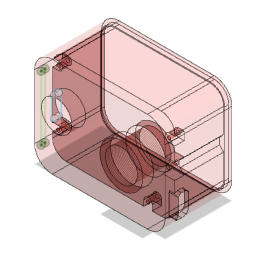
MDCEnclosure (Autodesk Fusion 360 design; units mm, degrees)
Autodesk Fusion 360 part; units mm, degrees
(part 1 of 2)
sketch "BackplateMountPoint" plane through (0, 0, 0) normal (0, 0, 1) x (1, 0, 0)
  line L0 (44.005, 19.075) -> (42.505, 17.575)
  line L1 (42.505, 17.575) -> (42.505, 15.075)
  line L2 (42.505, 15.075) -> (44.005, 13.575)
  line L3 (44.005, 13.575) -> (44.005, 19.075)
  line L4 (44.005, 16.325) -> (42.505, 16.325) construction
  line L5 (44.005, 4.75) -> (44.005, 27.9)
  point P0 (43.905, 16.325)
  dimension "d514" = 1.5
  dimension "d515" = 135
  dimension "d516" = 135
  dimension "d517" = 2.5
  dimension "d518" = 0.1
  constraint midpoint L3 L4.start
  constraint coincident L4 P0
  constraint midpoint L3 L5
  measures "d514" distance of L1 L3
  measures "d515" angle of L0 L1
  measures "d516" angle of L1 L2
  measures "d517" distance of L0.end L1.end
  measures "d518" distance of L3 P0
sketch "Board" plane through (0, 0, 0) normal (0, 0, 1) x (1, 0, 0)
  line L0 (4.75, 0) -> (39.105, 0)
  line L1 (43.855, 4.75) -> (43.855, 27.9)
  line L2 (39.105, 32.65) -> (4.75, 32.65)
  line L3 (0, 27.9) -> (0, 4.75)
  arc A0 (4.75, 32.65) -> (0, 27.9) centre (4.75, 27.9) ccw
  arc A1 (43.855, 27.9) -> (39.105, 32.65) centre (39.105, 27.9) ccw
  arc A2 (39.105, 0) -> (43.855, 4.75) centre (39.105, 4.75) ccw
  arc A3 (0, 4.75) -> (4.75, 0) centre (4.75, 4.75) ccw
  line L4 (-0.15, 27.9) -> (-0.15, 4.75)
  arc A4 (-0.15, 4.75) -> (4.75, -0.15) centre (4.75, 4.75) ccw
  line L5 (4.75, -0.15) -> (39.105, -0.15)
  arc A5 (39.105, -0.15) -> (44.005, 4.75) centre (39.105, 4.75) ccw
  line L6 (44.005, 4.75) -> (44.005, 27.9)
  arc A6 (44.005, 27.9) -> (39.105, 32.8) centre (39.105, 27.9) ccw
  line L7 (39.105, 32.8) -> (4.75, 32.8)
  arc A7 (4.75, 32.8) -> (-0.15, 27.9) centre (4.75, 27.9) ccw
  line L8 (-0.35, 27.9) -> (-0.35, 4.75)
  arc A8 (-0.35, 4.75) -> (4.75, -0.35) centre (4.75, 4.75) ccw
  line L9 (4.75, -0.35) -> (39.105, -0.35)
  arc A9 (39.105, -0.35) -> (44.205, 4.75) centre (39.105, 4.75) ccw
  line L10 (44.205, 4.75) -> (44.205, 27.9)
  arc A10 (44.205, 27.9) -> (39.105, 33) centre (39.105, 27.9) ccw
  line L11 (39.105, 33) -> (4.75, 33)
  arc A11 (4.75, 33) -> (-0.35, 27.9) centre (4.75, 27.9) ccw
  line L12 (-0.5, 27.9) -> (-0.5, 4.75)
  arc A12 (-0.5, 4.75) -> (4.75, -0.5) centre (4.75, 4.75) ccw
  line L13 (4.75, -0.5) -> (39.105, -0.5)
  arc A13 (39.105, -0.5) -> (44.355, 4.75) centre (39.105, 4.75) ccw
  line L14 (44.355, 4.75) -> (44.355, 27.9)
  arc A14 (44.355, 27.9) -> (39.105, 33.15) centre (39.105, 27.9) ccw
  line L15 (39.105, 33.15) -> (4.75, 33.15)
  arc A15 (4.75, 33.15) -> (-0.5, 27.9) centre (4.75, 27.9) ccw
  line L16 (21.9275, 32.65) -> (21.9275, 0)
  point P0 (21.9275, 16.325)
  dimension "d329" = 43.855
  dimension "d330" = 32.65
  dimension "d331" = 4.75
  dimension "d332" = 0.15
  dimension "d336" = 0.35
  dimension "d337" = 0.5
  constraint horizontal L0
  constraint vertical L1
  constraint horizontal L2
  constraint vertical L3
  constraint tangent L2 A0
  constraint tangent L3 A0
  constraint tangent L1 A1
  constraint tangent L2 A1
  constraint equal A0 A1
  constraint tangent L0 A2
  constraint tangent L1 A2
  constraint equal A0 A2
  constraint tangent L0 A3
  constraint tangent L3 A3
  constraint equal A0 A3
  constraint midpoint L2 L16.start
  constraint midpoint L0 L16.end
  constraint midpoint L16 P0
  measures "d329" distance of L1 L3
  measures "d330" distance of L0 L2
  measures "d331" radius of A0
sketch "MountPoints" plane through (0, 0, 0) normal (0, 0, 1) x (1, 0, 0)
  line L0 (-0.15, 29.9) -> (0.44, 29.9)
  line L1 (0.44, 29.9) -> (0.44, 26.9)
  line L2 (0.44, 26.9) -> (-0.15, 26.9)
  line L3 (-0.15, 26.9) -> (-0.15, 29.9)
  line L4 (0.44, 29.9) -> (1.94, 29.9)
  line L5 (3.44, 28.4) -> (3.44, 28.4)
  line L6 (1.94, 26.9) -> (0.44, 26.9)
  line L7 (0.44, 26.9) -> (0.44, 29.9)
  line L8 (43.472, 27.333) -> (44.005, 27.333)
  line L9 (44.005, 27.333) -> (44.005, 24.333)
  line L10 (44.005, 24.333) -> (43.472, 24.333)
  line L11 (43.472, 24.333) -> (43.472, 27.333)
  line L12 (41.972, 27.333) -> (43.472, 27.333)
  line L13 (43.472, 27.333) -> (43.472, 24.333)
  line L14 (43.472, 24.333) -> (41.972, 24.333)
  line L15 (40.472, 25.833) -> (40.472, 25.833)
  line L16 (34.3061, 3.4078) -> (34.3065, 3.4078)
  line L17 (35.8063, 1.9078) -> (35.8063, 0.4078)
  line L18 (35.8063, 0.4078) -> (32.8063, 0.4078)
  line L19 (32.8063, 0.4078) -> (32.8063, 1.9078)
  line L20 (32.8063, 0.4078) -> (35.8063, 0.4078)
  line L21 (35.8063, 0.4078) -> (35.8063, -0.15)
  line L22 (35.8063, -0.15) -> (32.8063, -0.15)
  line L23 (32.8063, -0.15) -> (32.8063, 0.4078)
  line L24 (0.39, 9.672) -> (1.89, 9.672)
  line L25 (3.39, 8.172) -> (3.39, 8.172)
  line L26 (1.89, 6.672) -> (0.39, 6.672)
  line L27 (0.39, 6.672) -> (0.39, 9.672)
  line L28 (-0.15, 9.672) -> (0.39, 9.672)
  line L29 (0.39, 9.672) -> (0.39, 6.672)
  line L30 (0.39, 6.672) -> (-0.15, 6.672)
  line L31 (-0.15, 6.672) -> (-0.15, 9.672)
  line L32 (-0.15, 27.9) -> (-0.15, 4.75)
  line L33 (44.005, 4.75) -> (44.005, 27.9)
  line L34 (4.75, -0.15) -> (39.105, -0.15)
  line L35 (0.44, 28.4) -> (3.44, 28.4) construction
  line L36 (40.472, 25.833) -> (43.472, 25.833) construction
  line L37 (32.8063, 1.9078) -> (35.8063, 1.9078) construction
  line L38 (0.39, 8.172) -> (3.39, 8.172) construction
  line L39 (0, 27.9) -> (0, 4.75) construction
  line L40 (4.75, 0) -> (39.105, 0) construction
  arc A0 (3.44, 28.4) -> (1.94, 29.9) centre (1.94, 28.4) ccw
  arc A1 (1.94, 26.9) -> (3.44, 28.4) centre (1.94, 28.4) ccw
  arc A2 (41.972, 27.333) -> (40.472, 25.833) centre (41.972, 25.833) ccw
  arc A3 (40.472, 25.833) -> (41.972, 24.333) centre (41.972, 25.833) ccw
  arc A4 (34.3061, 3.4078) -> (32.8063, 1.9078) centre (34.3063, 1.9078) ccw
  arc A5 (35.8063, 1.9078) -> (34.3065, 3.4078) centre (34.3063, 1.9078) ccw
  arc A6 (3.39, 8.172) -> (1.89, 9.672) centre (1.89, 8.172) ccw
  arc A7 (1.89, 6.672) -> (3.39, 8.172) centre (1.89, 8.172) ccw
  line L41 (44.005, 19.175) -> (39.505, 19.175)
  line L42 (39.505, 19.175) -> (39.505, 13.475)
  line L43 (39.505, 13.475) -> (44.005, 13.475)
  line L44 (44.005, 13.475) -> (44.005, 19.175)
  line L45 (44.005, 4.75) -> (44.005, 27.9)
  line L46 (44.005, 13.575) -> (44.005, 19.075)
  line L47 (44.005, 16.325) -> (39.505, 16.325)
  point P0 (1.94, 28.4)
  point P1 (41.972, 25.833)
  point P2 (34.3063, 1.9078)
  point P3 (1.89, 8.172)
  point P4 (44.005, 19.075)
  point P5 (41.505, 16.325)
  dimension "d404" = 3
  dimension "d407" = 3
  dimension "d409" = 3
  dimension "d411" = 3
  dimension "d412" = 1.89
  dimension "d413" = 8.172
  dimension "d414" = 34.3063
  dimension "d415" = 1.9078
  dimension "d416" = 41.972
  dimension "d417" = 25.833
  dimension "d418" = 1.94
  dimension "d419" = 28.4
  dimension "d422" = 1.5
  dimension "d566" = 0.1
  dimension "d567" = 4.5
  dimension "d568" = 2.5
  constraint horizontal L0
  constraint vertical L1
  constraint horizontal L2
  constraint vertical L3
  constraint horizontal L4
  constraint horizontal L6
  constraint vertical L7
  constraint horizontal L8
  constraint vertical L9
  constraint horizontal L10
  constraint vertical L11
  constraint horizontal L12
  constraint vertical L13
  constraint horizontal L14
  constraint vertical L17
  constraint horizontal L18
  constraint vertical L19
  constraint horizontal L20
  constraint vertical L21
  constraint horizontal L22
  constraint vertical L23
  constraint horizontal L24
  constraint horizontal L26
  constraint vertical L27
  constraint horizontal L28
  constraint vertical L29
  constraint horizontal L30
  constraint vertical L31
  constraint collinear L1 L7
  constraint collinear L0 L4
  constraint collinear L2 L6
  constraint collinear L3 L32
  constraint collinear L11 L13
  constraint collinear L9 L33
  constraint collinear L8 L12
  constraint collinear L10 L14
  constraint collinear L18 L20
  constraint collinear L22 L34
  constraint collinear L19 L23
  constraint collinear L17 L21
  constraint collinear L27 L29
  constraint collinear L24 L28
  constraint collinear L26 L30
  constraint collinear L31 L32
  constraint midpoint L1 L35.start
  constraint midpoint L13 L36.end
  constraint midpoint L29 L38.start
  constraint midpoint L35 P0
  constraint midpoint L36 P1
  constraint midpoint L37 P2
  constraint midpoint L38 P3
  constraint tangent L4 A0
  constraint tangent L6 A1
  constraint equal A0 A1
  constraint tangent L12 A2
  constraint equal A0 A2
  constraint tangent L14 A3
  constraint equal A0 A3
  constraint coincident L19 L37.start
  constraint tangent L19 A4
  constraint equal A0 A4
  constraint coincident L17 L37.end
  constraint tangent L17 A5
  constraint equal A0 A5
  constraint tangent L24 A6
  constraint equal A0 A6
  constraint tangent L26 A7
  constraint equal A0 A7
  constraint horizontal L41
  constraint vertical L42
  constraint horizontal L43
  constraint vertical L44
  constraint midpoint L44 L45
  constraint midpoint L46 L47.start
  constraint midpoint L42 L47.end
  constraint coincident L47 P5
  measures "d404" distance of L4 L6
  measures "d407" distance of L12 L14
  measures "d409" distance of L17 L19
  measures "d411" distance of L24 L26
  measures "d412" distance of P3 L39
  measures "d413" distance of P3 L40
  measures "d414" distance of P2 L39
  measures "d415" distance of P2 L40
  measures "d416" distance of P1 L39
  measures "d417" distance of P1 L40
  measures "d418" distance of P0 L39
  measures "d419" distance of P0 L40
  measures "d422" radius of A0
  measures "d566" distance of L41 P4
  measures "d567" distance of L42 L46
  measures "d568" distance of L44 P5
extrude "Front-Sidewalls" add sketch "Board" along normal blind 24.16 thin wall 1.5 on the left open curves L4 A4 L5 A5 L6 A6 L7 A7 makes body 1 in component "Front"
sketch "FrontHoles" plane through (0, 0, 0) normal (0, 0, 1) x (1, 0, 0)
  line L0 (0, 27.9) -> (0, 4.75)
  line L1 (4.75, 0) -> (39.105, 0)
  circle A0 centre (33.5424, 17.392) radius 7.2644
  circle A1 centre (33.5424, 17.392) radius 7.7644
  point P0 (6.2926, 17.392)
  point P1 (33.5424, 17.392)
  dimension "d350" = 6.2926
  dimension "d351" = 17.392
  dimension "d352" = 33.5424
  dimension "d353" = 17.392
  dimension "d554" = 14.5287
  dimension "d555" = 15.5287
  measures "d350" distance of P0 L0
  measures "d351" distance of P0 L1
  measures "d352" distance of P1 L0
  measures "d353" distance of P1 L1
  measures "d554" diameter of A0
  measures "d555" diameter of A1
extrude "Front-Frontplate" add sketch "Board" along normal blind 5 separate body contours L0 L2 L3 A0 A3 L16 | L0 L1 L2 A1 A2 L16 | L4 A4 L5 A5 L6 A6 L7 A7 makes body 2 in component "Front"
hole "Front-MotionSensorHole" at (6.2926, 17.392, 0) direction (0, 0, 1) diameter 11 depth 12 tip angle 118 bodies 2 in component "Front"
extrude "Front-LensProtrusionInside" [suppressed]
extrude "Extrude12" add sketch "FrontHoles" against normal blind 3.36 contours A0 bodies 2 in component "Front"
extrude "Front-LensProtrusionOutside" [suppressed]
extrude "Extrude13" add sketch "FrontHoles" along normal blind 8.84 contours A0 | A1 bodies 2 in component "Front"
hole "Hole8" at (33.5424, 17.392, -3.36) direction (0, 0, 1) diameter 11.529 end through all bodies 1 2 in component "Front"
thread "Thread2" "ISO Metric profile 12.0 M12x0.5 6H" major diameter 12.0961 minor diameter 11.5287 pitch 0.5 angle 60 resizes the face on face at (33.8297, 23.1493, 0.7067) on bodies 2 in component "Front"
copy_body "Body->Comp3" bodies 2 removing the originals makes body 3 in component "Component"
extrude "Front-BoardMountPoints" add sketch "MountPoints" against normal blind 3.36 separate body contours L0 L1 L2 L3 L7 L32 | L1 L4 L6 L7 A0 A1 | L8 L9 L10 L11 L13 L33 L45 | L11 L12 L13 L14 A2 A3 | L17 L18 L19 L20 A4 A5 | L18 L20 L21 L22 L23 L34 | L24 L26 L27 L29 A6 A7 | L27 L28 L29 L30 L31 L32 makes body 4 at (3.0647, 27.4075, -1.12) makes body 5 at (3.3895, 8.1346, -2.24) makes body 6 at (41.1898, 27.1129, -2.24) makes body 7 at (34.8063, -0.15, -1.12) in component "Component"
hole "Front-BoardMountPointHoles" at (41.972, 25.833, 0) at (1.94, 28.4, 0) at (1.89, 8.172, 0) at (34.3063, 1.9078, 0) direction (0, 0, -1) diameter 1.3 depth 3.36 tip angle 180 bodies 4 5 6 7 in component "Component"
extrude "Front-BackplateInset" cut sketch "Board" along normal blind 1.5 contours L0 L2 L3 A0 A3 L16 | L0 L1 L2 A1 A2 L16 | L4 A4 L5 A5 L6 A6 L7 A7 | L8 A8 L9 A9 L10 A10 L11 A11 | L12 A12 L13 A13 L14 A14 L15 A15 bodies 1 in component "Front"
extrude "Front-BackplateMountPoint" add sketch "BackplateMountPoint" along normal blind 19.16 from surface at 1.5 bodies 1 in component "Front"
move_body "Front-FrontplateAlign" bodies 6 4 3 7 5 to x (1, 0, 0) y (0, 1, 0) z (0, 0, 1) at (0, 0, 19.16) in component "Component"
extrude "Front-BackplateMountPointExtrude" add sketch "MountPoints" along normal blind 3.36 separate body contours L33 L42 L43 L44 L45 L46 L47 | L33 L41 L42 L44 L45 L46 L47 makes body 8 in component "Front"
hole "Hole9" at (41.505, 16.325, 0) direction (0, 0, 1) diameter 1.271 depth 3.36 tip angle 180 bodies 8 in component "Front"
thread "Thread3" "ISO Metric profile 1.6 M1.6x0.35 6H" in component "Front"
move_body "Front-BackplateMountPointAlign" bodies 8 to x (1, 0, 0) y (0, 1, 0) z (0, 0, 1) at (0, 0, 15.8) in component "Front"
combine "Front-Combine" operation add target body 1 tool bodies 3 4 7 5 6 8 in component "Front"
extrude "Back-Backplate" add sketch "Board" along normal blind 1.5 separate body contours L0 L2 L3 A0 A3 L16 | L0 L1 L2 A1 A2 L16 | L4 A4 L5 A5 L6 A6 L7 A7 | L8 A8 L9 A9 L10 A10 L11 A11 makes body 9 in component "Back"
sketch "HoleSemicircleTool" plane through (0, 0, 0) normal (0, 0, 1) x (1, 0, 0) in component "Back"
  line L0 (-2.65, 16.975) -> (-0.05, 16.975)
  line L1 (-0.05, 16.975) -> (-0.05, 15.675)
  line L2 (-0.05, 15.675) -> (-2.65, 15.675)
  line L3 (-2.65, 15.675) -> (-2.65, 16.975)
  point P0 (-0.05, 16.325)
  dimension "d509" = 1.3
  dimension "d510" = 2.6
  constraint horizontal L0
  constraint vertical L1
  constraint horizontal L2
  constraint vertical L3
  constraint midpoint L1 P0
  measures "d509" distance of L0 L2
  measures "d510" distance of L1 L3
extrude "Extrude3" cut sketch "HoleSemicircleTool" along normal blind 1.5 bodies 9 in component "Back"
sketch "Sketch1" plane through (0, 0, 0) normal (0, 0, 1) x (1, 0, 0) in component "Battery"
  line L0 (20, 15) -> (-20, 15)
  line L1 (-20, 15) -> (-20, -15)
  line L2 (-20, -15) -> (20, -15)
  line L3 (20, -15) -> (20, 15)
  line L4 (20, 15) -> (-20, -15) construction
  dimension "d443" = 40
  dimension "d444" = 30
  constraint horizontal L0
  constraint vertical L1
  constraint horizontal L2
  constraint vertical L3
  constraint midpoint L4 origin
  measures "d443" distance of L1 L3
  measures "d444" distance of L0 L2
extrude "Extrude1" add sketch "Sketch1" along normal blind 11.2 separate body makes body 10 in component "Battery"
move_body "Align1" bodies 10 to x (1, 0, 0) y (0, 1, 0) z (0, 0, 1) at (21.9275, 16.325, 1.5) in component "Battery"
ref_plane "WorkPlane3" through (21.9275, 16.325, 12.08) normal (1, 0, 0) x (0, 1, 0) in component "Front"
sketch "BackplateScrewHeadInset" plane through (0, 0, 0) normal (0, 0, 1) x (1, 0, 0)
  line L0 (0.45, 17.825) -> (-10.05, 17.825)
  line L1 (-10.05, 17.825) -> (-10.05, 14.825)
  line L2 (-10.05, 14.825) -> (0.45, 14.825)
  line L3 (1.45, 15.825) -> (1.45, 16.825)
  line L4 (1.45, 16.325) -> (-10.05, 16.325)
  arc A0 (1.45, 16.825) -> (0.45, 17.825) centre (0.45, 16.825) ccw
  arc A1 (0.45, 14.825) -> (1.45, 15.825) centre (0.45, 15.825) ccw
  point P0 (-0.05, 16.325)
  point P1 (-0.05, 16.325)
  dimension "d461" = 3
  dimension "d462" = 1.5
  dimension "d463" = 1
  dimension "d464" = 10
  constraint horizontal L0
  constraint vertical L1
  constraint horizontal L2
  constraint vertical L3
  constraint midpoint L1 L4.end
  constraint coincident L4 P1
  constraint coincident L3 L4.start
  constraint tangent L0 A0
  constraint tangent L3 A0
  constraint tangent L2 A1
  constraint tangent L3 A1
  constraint equal A0 A1
  constraint coincident P1 P0
  measures "d461" distance of L0 L2
  measures "d462" distance of L3 P1
  measures "d463" radius of A0
  measures "d464" distance of L1 P1
extrude "Extrude1'" add sketch "Board" along normal blind 3.1 separate body contours L0 L2 L3 A0 A3 L16 | L0 L1 L2 A1 A2 L16 makes body 11 in component "Board"
move_body "Align1'" bodies 11 to x (1, 0, 0) y (0, 1, 0) z (0, 0, 1) at (0, 0, 12.7) in component "Board"
sketch "USBCPlugCutout" plane through (0, 0, 0) normal (1, 0, 0) x (0, 0, -1) in component "Front"
  line L0 (-22, 4.75) -> (-22, 27.9)
  line L1 (-22, 27.9) -> (-23.5, 27.9)
  line L2 (-23.5, 27.9) -> (-23.5, 4.75)
  line L3 (-23.5, 4.75) -> (-22, 4.75)
  line L4 (-18.715, 19.0109) -> (-17.155, 19.0109)
  line L5 (-16.155, 18.0109) -> (-16.155, 10.6709)
  line L6 (-17.155, 9.6709) -> (-18.715, 9.6709)
  line L7 (-19.715, 10.6709) -> (-19.715, 18.0109)
  arc A0 (-18.715, 19.0109) -> (-19.715, 18.0109) centre (-18.715, 18.0109) ccw
  arc A1 (-16.155, 18.0109) -> (-17.155, 19.0109) centre (-17.155, 18.0109) ccw
  arc A2 (-17.155, 9.6709) -> (-16.155, 10.6709) centre (-17.155, 10.6709) ccw
  arc A3 (-19.715, 10.6709) -> (-18.715, 9.6709) centre (-18.715, 10.6709) ccw
  dimension "d492" = 3.56
  dimension "d493" = 9.34
  dimension "d497" = 1
  dimension "d498" = 1
  dimension "d499" = 1
  constraint horizontal L4
  constraint vertical L5
  constraint vertical L7
  constraint tangent L4 A0
  constraint tangent L7 A0
  constraint tangent L4 A1
  constraint tangent L5 A1
  constraint tangent L5 A2
  constraint tangent L6 A2
  constraint tangent L6 A3
  constraint tangent L7 A3
  constraint equal A2 A3
  measures "d492" distance of L5 L7
  measures "d493" distance of L4 L6
  measures "d497" radius of A0
  measures "d498" radius of A1
  measures "d499" radius of A2
extrude "Extrude9" add sketch "USBCPlugCutout" along normal blind 10 separate body contours L4 L5 L6 L7 A0 A1 A2 A3 makes body 12 in component "Front"
ref_plane "WorkPlane5" through (34.3063, 1.6289, 15.7) normal (0, 0, -1) x (-1, 0, 0) in component "Front"
ref_plane "WorkPlane6" through (42.005, 16.325, 21.66) normal (1, 0, 0) x (0, 1, 0) in component "Front"
move_body "Align3" bodies 12 to x (1, 0, 0) y (0, 1, 0) z (0, 0, 1) at (42.005, 0, 0) in component "Front"
move_body "Align4" bodies 12 to x (1, 0, 0) y (0, 1, 0) z (0, 0, 1) at (0, 0, -0.455) in component "Front"
ref_plane "WorkPlane7" through (21.9275, 0, 0) normal (0, -1, 0) x (1, 0, 0) in component "Front"
ref_plane "WorkPlane9" through (21.9275, 5.2535, 0) normal (0, -1, 0) x (1, 0, 0) in component "Front"
move_body "Align5" bodies 12 to x (1, 0, 0) y (0, 1, 0) z (0, 0, 1) at (0, -9.0874, 0) in component "Front"
combine "Combine3" operation cut target body 1 tool bodies 12 in component "Front"
sketch "MDC" plane through (0, 0, 0) normal (0, 0, 1) x (1, 0, 0) in component "PCB"
  arc A0 (41.5, 32.002) -> (39.105, 32.65) centre (39.105, 27.9) ccw
  line L0 (39.105, 32.65) -> (4.75, 32.65)
  arc A1 (39.105, 0) -> (43.855, 4.75) centre (39.105, 4.75) ccw
  line L1 (0, 27.9) -> (0, 4.75)
  line L2 (43.855, 4.75) -> (43.855, 27.94)
  arc A2 (0, 4.75) -> (4.75, 0) centre (4.75, 4.75) ccw
  circle A3 centre (33.5424, 26.392) radius 0.85
  line L3 (41.5, 27.94) -> (41.5, 32.002)
  line L4 (4.75, 0) -> (39.105, 0)
  line L5 (41.5, 27.94) -> (43.855, 27.94)
  arc A4 (4.75, 32.65) -> (0, 27.9) centre (4.75, 27.9) ccw
  circle A5 centre (33.5424, 8.392) radius 0.85
  circle A6 centre (31.327, 4.655) radius 0.4953
  arc A7 (20.7054, 5.534) -> (20.7054, 5.7626) centre (20.7054, 5.6483) ccw
  arc A8 (20.7054, 5.534) -> (20.7054, 5.7626) centre (20.7054, 5.6483) ccw
  arc A9 (20.7054, 5.7626) -> (20.7054, 5.534) centre (20.7054, 5.6483) ccw
  arc A10 (20.7054, 5.7626) -> (20.7054, 5.534) centre (20.7054, 5.6483) ccw
  arc A11 (25.253, 5.5373) -> (25.253, 5.7659) centre (25.253, 5.6516) ccw
  arc A12 (25.253, 5.7659) -> (25.253, 5.5373) centre (25.253, 5.6516) ccw
  arc A13 (24.6078, 4.8871) -> (24.6078, 5.1157) centre (24.6078, 5.0014) ccw
  arc A14 (21.5834, 17.8471) -> (21.5834, 18.0757) centre (21.5834, 17.9614) ccw
  arc A15 (1.89, 8.922) -> (1.89, 7.422) centre (1.89, 8.172) ccw
  arc A16 (21.5834, 17.8471) -> (21.5834, 18.0757) centre (21.5834, 17.9614) ccw
  arc A17 (21.5834, 18.0757) -> (21.5834, 17.8471) centre (21.5834, 17.9614) ccw
  arc A18 (21.5834, 17.0597) -> (21.5834, 17.2883) centre (21.5834, 17.174) ccw
  arc A19 (21.5834, 18.0757) -> (21.5834, 17.8471) centre (21.5834, 17.9614) ccw
  arc A20 (20.7706, 17.0597) -> (20.7706, 17.2883) centre (20.7706, 17.174) ccw
  arc A21 (20.7706, 17.2883) -> (20.7706, 17.0597) centre (20.7706, 17.174) ccw
  arc A22 (20.7706, 16.2469) -> (20.7706, 16.4755) centre (20.7706, 16.3612) ccw
  arc A23 (21.5834, 17.2883) -> (21.5834, 17.0597) centre (21.5834, 17.174) ccw
  arc A24 (21.5834, 17.2883) -> (21.5834, 17.0597) centre (21.5834, 17.174) ccw
  arc A25 (21.5834, 17.0597) -> (21.5834, 17.2883) centre (21.5834, 17.174) ccw
  arc A26 (25.2581, 4.8896) -> (25.2581, 5.1182) centre (25.2581, 5.0039) ccw
  arc A27 (25.2581, 5.1182) -> (25.2581, 4.8896) centre (25.2581, 5.0039) ccw
  arc A28 (25.2581, 4.8896) -> (25.2581, 5.1182) centre (25.2581, 5.0039) ccw
  arc A29 (20.7706, 17.2883) -> (20.7706, 17.0597) centre (20.7706, 17.174) ccw
  arc A30 (20.7706, 17.0597) -> (20.7706, 17.2883) centre (20.7706, 17.174) ccw
  arc A31 (20.7706, 16.4755) -> (20.7706, 16.2469) centre (20.7706, 16.3612) ccw
  arc A32 (21.3566, 4.2368) -> (21.3566, 4.4654) centre (21.3566, 4.3511) ccw
  arc A33 (21.3566, 4.4654) -> (21.3566, 4.2368) centre (21.3566, 4.3511) ccw
  arc A34 (21.3566, 4.2368) -> (21.3566, 4.4654) centre (21.3566, 4.3511) ccw
  arc A35 (20.7706, 16.4755) -> (20.7706, 16.2469) centre (20.7706, 16.3612) ccw
  arc A36 (20.7706, 16.2469) -> (20.7706, 16.4755) centre (20.7706, 16.3612) ccw
  arc A37 (25.2581, 5.1182) -> (25.2581, 4.8896) centre (25.2581, 5.0039) ccw
  arc A38 (10.8138, 28.8136) -> (10.8138, 29.1057) centre (10.8138, 28.9596) ccw
  arc A39 (10.8138, 29.1057) -> (10.8138, 28.8136) centre (10.8138, 28.9596) ccw
  arc A40 (11.2431, 28.364) -> (11.2431, 28.6561) centre (11.2431, 28.51) ccw
  arc A41 (25.253, 5.7659) -> (25.253, 5.5373) centre (25.253, 5.6516) ccw
  arc A42 (25.253, 5.5373) -> (25.253, 5.7659) centre (25.253, 5.6516) ccw
  arc A43 (24.6078, 5.1157) -> (24.6078, 4.8871) centre (24.6078, 5.0014) ccw
  arc A44 (14.5578, 25.1534) -> (14.5578, 25.4455) centre (14.5578, 25.2995) ccw
  arc A45 (14.5578, 25.4455) -> (14.5578, 25.1534) centre (14.5578, 25.2995) ccw
  arc A46 (14.5578, 25.1534) -> (14.5578, 25.4455) centre (14.5578, 25.2995) ccw
  arc A47 (24.6078, 5.1157) -> (24.6078, 4.8871) centre (24.6078, 5.0014) ccw
  arc A48 (24.6078, 4.8871) -> (24.6078, 5.1157) centre (24.6078, 5.0014) ccw
  arc A49 (21.3566, 4.4654) -> (21.3566, 4.2368) centre (21.3566, 4.3511) ccw
  arc A50 (15.0556, 24.6988) -> (15.0556, 24.9908) centre (15.0556, 24.8448) ccw
  arc A51 (15.0556, 24.9908) -> (15.0556, 24.6988) centre (15.0556, 24.8448) ccw
  arc A52 (9.0891, 27.1804) -> (9.0891, 27.4724) centre (9.0891, 27.3264) ccw
  arc A53 (10.8138, 29.1057) -> (10.8138, 28.8136) centre (10.8138, 28.9596) ccw
  arc A54 (10.8138, 28.8136) -> (10.8138, 29.1057) centre (10.8138, 28.9596) ccw
  arc A55 (11.2431, 28.6561) -> (11.2431, 28.364) centre (11.2431, 28.51) ccw
  arc A56 (10.0569, 25.617) -> (10.0569, 25.8456) centre (10.0569, 25.7313) ccw
  arc A57 (10.0569, 25.8456) -> (10.0569, 25.617) centre (10.0569, 25.7313) ccw
  arc A58 (10.0569, 25.617) -> (10.0569, 25.8456) centre (10.0569, 25.7313) ccw
  arc A59 (11.2431, 28.6561) -> (11.2431, 28.364) centre (11.2431, 28.51) ccw
  arc A60 (11.2431, 28.364) -> (11.2431, 28.6561) centre (11.2431, 28.51) ccw
  arc A61 (14.5578, 25.4455) -> (14.5578, 25.1534) centre (14.5578, 25.2995) ccw
  arc A62 (11.1999, 24.479) -> (11.1999, 24.7076) centre (11.1999, 24.5933) ccw
  arc A63 (11.1999, 24.7076) -> (11.1999, 24.479) centre (11.1999, 24.5933) ccw
  arc A64 (12.8864, 21.6444) -> (12.8864, 21.873) centre (12.8864, 21.7587) ccw
  arc A65 (15.0556, 24.9908) -> (15.0556, 24.6988) centre (15.0556, 24.8448) ccw
  arc A66 (15.0556, 24.6988) -> (15.0556, 24.9908) centre (15.0556, 24.8448) ccw
  arc A67 (9.0891, 27.4724) -> (9.0891, 27.1804) centre (9.0891, 27.3264) ccw
  arc A68 (12.287, 28.9977) -> (12.287, 29.2263) centre (12.287, 29.112) ccw
  arc A69 (12.287, 29.2263) -> (12.287, 28.9977) centre (12.287, 29.112) ccw
  arc A70 (12.287, 28.9977) -> (12.287, 29.2263) centre (12.287, 29.112) ccw
  arc A71 (9.0891, 27.4724) -> (9.0891, 27.1804) centre (9.0891, 27.3264) ccw
  arc A72 (9.0891, 27.1804) -> (9.0891, 27.4724) centre (9.0891, 27.3264) ccw
  arc A73 (10.0569, 25.8456) -> (10.0569, 25.617) centre (10.0569, 25.7313) ccw
  arc A74 (13.4452, 27.8572) -> (13.4452, 28.0858) centre (13.4452, 27.9715) ccw
  arc A75 (13.4452, 28.0858) -> (13.4452, 27.8572) centre (13.4452, 27.9715) ccw
  arc A76 (12.2819, 24.446) -> (12.2819, 24.6746) centre (12.2819, 24.5603) ccw
  arc A77 (11.1999, 24.7076) -> (11.1999, 24.479) centre (11.1999, 24.5933) ccw
  arc A78 (11.1999, 24.479) -> (11.1999, 24.7076) centre (11.1999, 24.5933) ccw
  arc A79 (12.8864, 21.873) -> (12.8864, 21.6444) centre (12.8864, 21.7587) ccw
  arc A80 (14.0371, 26.2012) -> (14.0371, 26.4298) centre (14.0371, 26.3155) ccw
  arc A81 (14.0371, 26.4298) -> (14.0371, 26.2012) centre (14.0371, 26.3155) ccw
  arc A82 (14.0371, 26.2012) -> (14.0371, 26.4298) centre (14.0371, 26.3155) ccw
  arc A83 (12.8864, 21.873) -> (12.8864, 21.6444) centre (12.8864, 21.7587) ccw
  arc A84 (12.8864, 21.6444) -> (12.8864, 21.873) centre (12.8864, 21.7587) ccw
  arc A85 (12.287, 29.2263) -> (12.287, 28.9977) centre (12.287, 29.112) ccw
  arc A86 (6.9597, 9.5923) -> (6.9597, 9.8845) centre (6.9597, 9.7384) ccw
  arc A87 (6.9597, 9.8845) -> (6.9597, 9.5923) centre (6.9597, 9.7384) ccw
  arc A88 (6.9466, 8.9396) -> (6.9466, 9.2316) centre (6.9466, 9.0856) ccw
  arc A89 (13.4452, 28.0858) -> (13.4452, 27.8572) centre (13.4452, 27.9715) ccw
  arc A90 (13.4452, 27.8572) -> (13.4452, 28.0858) centre (13.4452, 27.9715) ccw
  arc A91 (12.2819, 24.6746) -> (12.2819, 24.446) centre (12.2819, 24.5603) ccw
  arc A92 (4.3625, 26.4779) -> (4.3625, 26.77) centre (4.3625, 26.6239) ccw
  arc A93 (4.3625, 26.77) -> (4.3625, 26.4779) centre (4.3625, 26.6239) ccw
  arc A94 (4.3625, 26.4779) -> (4.3625, 26.77) centre (4.3625, 26.6239) ccw
  arc A95 (12.2819, 24.6746) -> (12.2819, 24.446) centre (12.2819, 24.5603) ccw
  arc A96 (12.2819, 24.446) -> (12.2819, 24.6746) centre (12.2819, 24.5603) ccw
  arc A97 (14.0371, 26.4298) -> (14.0371, 26.2012) centre (14.0371, 26.3155) ccw
  arc A98 (19.6911, 6.487) -> (19.6911, 6.779) centre (19.6911, 6.633) ccw
  arc A99 (19.6911, 6.779) -> (19.6911, 6.487) centre (19.6911, 6.633) ccw
  arc A100 (23.9481, 7.1169) -> (23.9481, 7.409) centre (23.9481, 7.2629) ccw
  arc A101 (6.9597, 9.8845) -> (6.9597, 9.5923) centre (6.9597, 9.7384) ccw
  arc A102 (6.9597, 9.5923) -> (6.9597, 9.8845) centre (6.9597, 9.7384) ccw
  arc A103 (6.9466, 9.2316) -> (6.9466, 8.9396) centre (6.9466, 9.0856) ccw
  arc A104 (27.7556, 13.3538) -> (27.7556, 13.5824) centre (27.7556, 13.4681) ccw
  arc A105 (27.7556, 13.5824) -> (27.7556, 13.3538) centre (27.7556, 13.4681) ccw
  arc A106 (27.7556, 13.3538) -> (27.7556, 13.5824) centre (27.7556, 13.4681) ccw
  arc A107 (6.9466, 9.2316) -> (6.9466, 8.9396) centre (6.9466, 9.0856) ccw
  arc A108 (6.9466, 8.9396) -> (6.9466, 9.2316) centre (6.9466, 9.0856) ccw
  arc A109 (4.3625, 26.77) -> (4.3625, 26.4779) centre (4.3625, 26.6239) ccw
  arc A110 (27.7454, 12.6452) -> (27.7454, 12.8738) centre (27.7454, 12.7595) ccw
  arc A111 (27.7454, 12.8738) -> (27.7454, 12.6452) centre (27.7454, 12.7595) ccw
  arc A112 (17.8394, 3.8517) -> (17.8394, 4.0803) centre (17.8394, 3.966) ccw
  arc A113 (19.6911, 6.779) -> (19.6911, 6.487) centre (19.6911, 6.633) ccw
  arc A114 (19.6911, 6.487) -> (19.6911, 6.779) centre (19.6911, 6.633) ccw
  arc A115 (23.9481, 7.409) -> (23.9481, 7.1169) centre (23.9481, 7.2629) ccw
  arc A116 (20.7655, 15.4747) -> (20.7655, 15.7033) centre (20.7655, 15.589) ccw
  arc A117 (20.7655, 15.7033) -> (20.7655, 15.4747) centre (20.7655, 15.589) ccw
  arc A118 (20.7655, 15.4747) -> (20.7655, 15.7033) centre (20.7655, 15.589) ccw
  arc A119 (23.9481, 7.409) -> (23.9481, 7.1169) centre (23.9481, 7.2629) ccw
  arc A120 (23.9481, 7.1169) -> (23.9481, 7.409) centre (23.9481, 7.2629) ccw
  arc A121 (27.7556, 13.5824) -> (27.7556, 13.3538) centre (27.7556, 13.4681) ccw
  arc A122 (13.4275, 22.2235) -> (13.4275, 22.4521) centre (13.4275, 22.3378) ccw
  arc A123 (13.4275, 22.4521) -> (13.4275, 22.2235) centre (13.4275, 22.3378) ccw
  arc A124 (16.8893, 2.2531) -> (16.8893, 2.4817) centre (16.8893, 2.3674) ccw
  arc A125 (27.7454, 12.8738) -> (27.7454, 12.6452) centre (27.7454, 12.7595) ccw
  arc A126 (27.7454, 12.6452) -> (27.7454, 12.8738) centre (27.7454, 12.7595) ccw
  arc A127 (17.8394, 4.0803) -> (17.8394, 3.8517) centre (17.8394, 3.966) ccw
  arc A128 (16.8893, 5.5334) -> (16.8893, 5.762) centre (16.8893, 5.6477) ccw
  arc A129 (16.8893, 5.762) -> (16.8893, 5.5334) centre (16.8893, 5.6477) ccw
  arc A130 (16.8893, 5.5334) -> (16.8893, 5.762) centre (16.8893, 5.6477) ccw
  arc A131 (17.8394, 4.0803) -> (17.8394, 3.8517) centre (17.8394, 3.966) ccw
  arc A132 (17.8394, 3.8517) -> (17.8394, 4.0803) centre (17.8394, 3.966) ccw
  arc A133 (20.7655, 15.7033) -> (20.7655, 15.4747) centre (20.7655, 15.589) ccw
  arc A134 (11.4969, 5.912) -> (11.4969, 6.204) centre (11.4969, 6.058) ccw
  arc A135 (11.4969, 6.204) -> (11.4969, 5.912) centre (11.4969, 6.058) ccw
  arc A136 (28.543, 12.456) -> (28.543, 12.7481) centre (28.543, 12.602) ccw
  arc A137 (13.4275, 22.4521) -> (13.4275, 22.2235) centre (13.4275, 22.3378) ccw
  arc A138 (13.4275, 22.2235) -> (13.4275, 22.4521) centre (13.4275, 22.3378) ccw
  arc A139 (16.8893, 2.4817) -> (16.8893, 2.2531) centre (16.8893, 2.3674) ccw
  arc A140 (26.1224, 10.2514) -> (26.1224, 10.48) centre (26.1224, 10.3657) ccw
  arc A141 (26.1224, 10.48) -> (26.1224, 10.2514) centre (26.1224, 10.3657) ccw
  arc A142 (26.1224, 10.2514) -> (26.1224, 10.48) centre (26.1224, 10.3657) ccw
  arc A143 (16.8893, 2.4817) -> (16.8893, 2.2531) centre (16.8893, 2.3674) ccw
  arc A144 (16.8893, 2.2531) -> (16.8893, 2.4817) centre (16.8893, 2.3674) ccw
  arc A145 (16.8893, 5.762) -> (16.8893, 5.5334) centre (16.8893, 5.6477) ccw
  arc A146 (27.1333, 27.8155) -> (27.1333, 28.0441) centre (27.1333, 27.9298) ccw
  arc A147 (27.1333, 28.0441) -> (27.1333, 27.8155) centre (27.1333, 27.9298) ccw
  arc A148 (28.9011, 30.0711) -> (28.9011, 30.2997) centre (28.9011, 30.1854) ccw
  arc A149 (11.4969, 6.204) -> (11.4969, 5.912) centre (11.4969, 6.058) ccw
  arc A150 (11.4969, 5.912) -> (11.4969, 6.204) centre (11.4969, 6.058) ccw
  arc A151 (28.543, 12.7481) -> (28.543, 12.456) centre (28.543, 12.602) ccw
  arc A152 (28.416, 14.1097) -> (28.416, 14.3383) centre (28.416, 14.224) ccw
  arc A153 (28.416, 14.3383) -> (28.416, 14.1097) centre (28.416, 14.224) ccw
  arc A154 (28.416, 14.1097) -> (28.416, 14.3383) centre (28.416, 14.224) ccw
  arc A155 (28.543, 12.7481) -> (28.543, 12.456) centre (28.543, 12.602) ccw
  arc A156 (28.543, 12.456) -> (28.543, 12.7481) centre (28.543, 12.602) ccw
  arc A157 (26.1224, 10.48) -> (26.1224, 10.2514) centre (26.1224, 10.3657) ccw
  arc A158 (6.2824, 4.5644) -> (6.2824, 4.793) centre (6.2824, 4.6787) ccw
  arc A159 (6.2824, 4.793) -> (6.2824, 4.5644) centre (6.2824, 4.6787) ccw
  arc A160 (6.2824, 2.1844) -> (6.2824, 2.413) centre (6.2824, 2.2987) ccw
  arc A161 (27.1333, 28.0441) -> (27.1333, 27.8155) centre (27.1333, 27.9298) ccw
  arc A162 (27.1333, 27.8155) -> (27.1333, 28.0441) centre (27.1333, 27.9298) ccw
  arc A163 (28.9011, 30.2997) -> (28.9011, 30.0711) centre (28.9011, 30.1854) ccw
  arc A164 (27.2212, 19.0045) -> (27.2212, 19.2965) centre (27.2212, 19.1505) ccw
  arc A165 (27.2212, 19.2965) -> (27.2212, 19.0045) centre (27.2212, 19.1505) ccw
  arc A166 (27.2212, 19.0045) -> (27.2212, 19.2965) centre (27.2212, 19.1505) ccw
  arc A167 (28.9011, 30.2997) -> (28.9011, 30.0711) centre (28.9011, 30.1854) ccw
  arc A168 (28.9011, 30.0711) -> (28.9011, 30.2997) centre (28.9011, 30.1854) ccw
  arc A169 (28.416, 14.3383) -> (28.416, 14.1097) centre (28.416, 14.224) ccw
  arc A170 (18.51, 10.0457) -> (18.51, 10.2743) centre (18.51, 10.16) ccw
  arc A171 (18.51, 10.2743) -> (18.51, 10.0457) centre (18.51, 10.16) ccw
  arc A172 (17.9182, 6.2459) -> (17.9182, 6.4745) centre (17.9182, 6.3602) ccw
  arc A173 (6.2824, 4.793) -> (6.2824, 4.5644) centre (6.2824, 4.6787) ccw
  arc A174 (6.2824, 4.5644) -> (6.2824, 4.793) centre (6.2824, 4.6787) ccw
  arc A175 (6.2824, 2.413) -> (6.2824, 2.1844) centre (6.2824, 2.2987) ccw
  arc A176 (33.1074, 14.8996) -> (33.1074, 15.1282) centre (33.1074, 15.0139) ccw
  arc A177 (33.1074, 15.1282) -> (33.1074, 14.8996) centre (33.1074, 15.0139) ccw
  arc A178 (33.1074, 14.8996) -> (33.1074, 15.1282) centre (33.1074, 15.0139) ccw
  arc A179 (6.2824, 2.413) -> (6.2824, 2.1844) centre (6.2824, 2.2987) ccw
  arc A180 (6.2824, 2.1844) -> (6.2824, 2.413) centre (6.2824, 2.2987) ccw
  arc A181 (27.2212, 19.2965) -> (27.2212, 19.0045) centre (27.2212, 19.1505) ccw
  arc A182 (36.1224, 31.6954) -> (36.1224, 31.9874) centre (36.1224, 31.8414) ccw
  arc A183 (36.1224, 31.9874) -> (36.1224, 31.6954) centre (36.1224, 31.8414) ccw
  arc A184 (34.7609, 31.8846) -> (34.7609, 32.1132) centre (34.7609, 31.9989) ccw
  arc A185 (18.51, 10.2743) -> (18.51, 10.0457) centre (18.51, 10.16) ccw
  arc A186 (18.51, 10.0457) -> (18.51, 10.2743) centre (18.51, 10.16) ccw
  arc A187 (17.9182, 6.4745) -> (17.9182, 6.2459) centre (17.9182, 6.3602) ccw
  arc A188 (28.1849, 20.6654) -> (28.1849, 20.894) centre (28.1849, 20.7797) ccw
  arc A189 (28.1849, 20.894) -> (28.1849, 20.6654) centre (28.1849, 20.7797) ccw
  arc A190 (28.1849, 20.6654) -> (28.1849, 20.894) centre (28.1849, 20.7797) ccw
  arc A191 (17.9182, 6.4745) -> (17.9182, 6.2459) centre (17.9182, 6.3602) ccw
  arc A192 (17.9182, 6.2459) -> (17.9182, 6.4745) centre (17.9182, 6.3602) ccw
  arc A193 (33.1074, 15.1282) -> (33.1074, 14.8996) centre (33.1074, 15.0139) ccw
  arc A194 (29.526, 21.3563) -> (29.526, 21.5849) centre (29.526, 21.4706) ccw
  arc A195 (29.526, 21.5849) -> (29.526, 21.3563) centre (29.526, 21.4706) ccw
  arc A196 (30.2448, 4.0259) -> (30.2448, 4.2545) centre (30.2448, 4.1402) ccw
  arc A197 (36.1224, 31.9874) -> (36.1224, 31.6954) centre (36.1224, 31.8414) ccw
  arc A198 (36.1224, 31.6954) -> (36.1224, 31.9874) centre (36.1224, 31.8414) ccw
  arc A199 (34.7609, 32.1132) -> (34.7609, 31.8846) centre (34.7609, 31.9989) ccw
  arc A200 (30.0518, 2.601) -> (30.0518, 2.8296) centre (30.0518, 2.7153) ccw
  arc A201 (30.0518, 2.8296) -> (30.0518, 2.601) centre (30.0518, 2.7153) ccw
  arc A202 (30.0518, 2.601) -> (30.0518, 2.8296) centre (30.0518, 2.7153) ccw
  arc A203 (34.7609, 32.1132) -> (34.7609, 31.8846) centre (34.7609, 31.9989) ccw
  arc A204 (34.7609, 31.8846) -> (34.7609, 32.1132) centre (34.7609, 31.9989) ccw
  arc A205 (28.1849, 20.894) -> (28.1849, 20.6654) centre (28.1849, 20.7797) ccw
  arc A206 (13.2852, 6.2763) -> (13.2852, 6.5049) centre (13.2852, 6.3906) ccw
  arc A207 (13.2852, 6.5049) -> (13.2852, 6.2763) centre (13.2852, 6.3906) ccw
  arc A208 (12.7417, 5.4381) -> (12.7417, 5.6667) centre (12.7417, 5.5524) ccw
  arc A209 (29.526, 21.5849) -> (29.526, 21.3563) centre (29.526, 21.4706) ccw
  arc A210 (29.526, 21.3563) -> (29.526, 21.5849) centre (29.526, 21.4706) ccw
  arc A211 (30.2448, 4.2545) -> (30.2448, 4.0259) centre (30.2448, 4.1402) ccw
  arc A212 (9.7419, 5.9563) -> (9.7419, 6.1849) centre (9.7419, 6.0706) ccw
  arc A213 (9.7419, 6.1849) -> (9.7419, 5.9563) centre (9.7419, 6.0706) ccw
  arc A214 (9.7419, 5.9563) -> (9.7419, 6.1849) centre (9.7419, 6.0706) ccw
  arc A215 (30.2448, 4.2545) -> (30.2448, 4.0259) centre (30.2448, 4.1402) ccw
  arc A216 (30.2448, 4.0259) -> (30.2448, 4.2545) centre (30.2448, 4.1402) ccw
  arc A217 (30.0518, 2.8296) -> (30.0518, 2.601) centre (30.0518, 2.7153) ccw
  arc A218 (24.7508, 19.4437) -> (24.7508, 19.6723) centre (24.7508, 19.558) ccw
  arc A219 (24.7508, 19.6723) -> (24.7508, 19.4437) centre (24.7508, 19.558) ccw
  arc A220 (28.731, 23.4467) -> (28.731, 23.6753) centre (28.731, 23.561) ccw
  arc A221 (13.2852, 6.5049) -> (13.2852, 6.2763) centre (13.2852, 6.3906) ccw
  arc A222 (13.2852, 6.2763) -> (13.2852, 6.5049) centre (13.2852, 6.3906) ccw
  arc A223 (12.7417, 5.6667) -> (12.7417, 5.4381) centre (12.7417, 5.5524) ccw
  arc A224 (34.5222, 5.1392) -> (34.5222, 5.3678) centre (34.5222, 5.2535) ccw
  arc A225 (34.5222, 5.3678) -> (34.5222, 5.1392) centre (34.5222, 5.2535) ccw
  arc A226 (34.5222, 5.1392) -> (34.5222, 5.3678) centre (34.5222, 5.2535) ccw
  arc A227 (12.7417, 5.6667) -> (12.7417, 5.4381) centre (12.7417, 5.5524) ccw
  arc A228 (12.7417, 5.4381) -> (12.7417, 5.6667) centre (12.7417, 5.5524) ccw
  arc A229 (9.7419, 6.1849) -> (9.7419, 5.9563) centre (9.7419, 6.0706) ccw
  arc A230 (26.4983, 24.3916) -> (26.4983, 24.6202) centre (26.4983, 24.5059) ccw
  arc A231 (26.4983, 24.6202) -> (26.4983, 24.3916) centre (26.4983, 24.5059) ccw
  arc A232 (23.91, 28.9826) -> (23.91, 29.2747) centre (23.91, 29.1287) ccw
  arc A233 (24.7508, 19.6723) -> (24.7508, 19.4437) centre (24.7508, 19.558) ccw
  arc A234 (24.7508, 19.4437) -> (24.7508, 19.6723) centre (24.7508, 19.558) ccw
  arc A235 (28.731, 23.6753) -> (28.731, 23.4467) centre (28.731, 23.561) ccw
  arc A236 (32.226, 28.556) -> (32.226, 28.8481) centre (32.226, 28.702) ccw
  arc A237 (32.226, 28.8481) -> (32.226, 28.556) centre (32.226, 28.702) ccw
  arc A238 (32.226, 28.556) -> (32.226, 28.8481) centre (32.226, 28.702) ccw
  arc A239 (28.731, 23.6753) -> (28.731, 23.4467) centre (28.731, 23.561) ccw
  arc A240 (28.731, 23.4467) -> (28.731, 23.6753) centre (28.731, 23.561) ccw
  arc A241 (34.5222, 5.3678) -> (34.5222, 5.1392) centre (34.5222, 5.2535) ccw
  arc A242 (28.7919, 26.3601) -> (28.7919, 26.5887) centre (28.7919, 26.4744) ccw
  arc A243 (28.7919, 26.5887) -> (28.7919, 26.3601) centre (28.7919, 26.4744) ccw
  arc A244 (36.29, 13.5699) -> (36.29, 13.862) centre (36.29, 13.716) ccw
  arc A245 (26.4983, 24.6202) -> (26.4983, 24.3916) centre (26.4983, 24.5059) ccw
  arc A246 (26.4983, 24.3916) -> (26.4983, 24.6202) centre (26.4983, 24.5059) ccw
  arc A247 (23.91, 29.2747) -> (23.91, 28.9826) centre (23.91, 29.1287) ccw
  arc A248 (36.29, 12.808) -> (36.29, 13.1) centre (36.29, 12.954) ccw
  arc A249 (36.29, 13.1) -> (36.29, 12.808) centre (36.29, 12.954) ccw
  arc A250 (36.29, 12.808) -> (36.29, 13.1) centre (36.29, 12.954) ccw
  arc A251 (23.91, 29.2747) -> (23.91, 28.9826) centre (23.91, 29.1287) ccw
  arc A252 (23.91, 28.9826) -> (23.91, 29.2747) centre (23.91, 29.1287) ccw
  arc A253 (32.226, 28.8481) -> (32.226, 28.556) centre (32.226, 28.702) ccw
  arc A254 (30.9306, 16.7869) -> (30.9306, 17.0155) centre (30.9306, 16.9012) ccw
  arc A255 (30.9306, 17.0155) -> (30.9306, 16.7869) centre (30.9306, 16.9012) ccw
  arc A256 (28.7919, 26.5887) -> (28.7919, 26.3601) centre (28.7919, 26.4744) ccw
  arc A257 (28.7919, 26.3601) -> (28.7919, 26.5887) centre (28.7919, 26.4744) ccw
  arc A258 (36.29, 13.862) -> (36.29, 13.5699) centre (36.29, 13.716) ccw
  arc A259 (10.6858, 8.7122) -> (10.6858, 8.9408) centre (10.6858, 8.8265) ccw
  arc A260 (10.6858, 8.9408) -> (10.6858, 8.7122) centre (10.6858, 8.8265) ccw
  arc A261 (36.29, 13.862) -> (36.29, 13.5699) centre (36.29, 13.716) ccw
  arc A262 (36.29, 13.5699) -> (36.29, 13.862) centre (36.29, 13.716) ccw
  arc A263 (36.29, 13.1) -> (36.29, 12.808) centre (36.29, 12.954) ccw
  arc A264 (1.89, 7.422) -> (1.89, 8.922) centre (1.89, 8.172) ccw
  arc A265 (1.89, 7.422) -> (1.89, 8.922) centre (1.89, 8.172) ccw
  arc A266 (30.9306, 17.0155) -> (30.9306, 16.7869) centre (30.9306, 16.9012) ccw
  arc A267 (30.9306, 16.7869) -> (30.9306, 17.0155) centre (30.9306, 16.9012) ccw
  arc A268 (1.94, 27.65) -> (1.94, 29.15) centre (1.94, 28.4) ccw
  arc A269 (1.94, 27.65) -> (1.94, 29.15) centre (1.94, 28.4) ccw
  arc A270 (1.89, 8.922) -> (1.89, 7.422) centre (1.89, 8.172) ccw
  arc A271 (1.94, 29.15) -> (1.94, 27.65) centre (1.94, 28.4) ccw
  arc A272 (41.7272, 10.9338) -> (41.7272, 11.2104) centre (41.7272, 11.0721) ccw
  arc A273 (34.3063, 1.1578) -> (34.3063, 2.6578) centre (34.3063, 1.9078) ccw
  arc A274 (34.3063, 1.1578) -> (34.3063, 2.6578) centre (34.3063, 1.9078) ccw
  arc A275 (41.972, 25.083) -> (41.972, 26.583) centre (41.972, 25.833) ccw
  arc A276 (1.94, 29.15) -> (1.94, 27.65) centre (1.94, 28.4) ccw
  arc A277 (41.972, 25.083) -> (41.972, 26.583) centre (41.972, 25.833) ccw
  arc A278 (41.7272, 11.2104) -> (41.7272, 10.9338) centre (41.7272, 11.0721) ccw
  arc A279 (41.7272, 11.2104) -> (41.7272, 10.9338) centre (41.7272, 11.0721) ccw
  arc A280 (39.5249, 2.2377) -> (39.5249, 2.4663) centre (39.5249, 2.352) ccw
  arc A281 (41.7272, 10.9338) -> (41.7272, 11.2104) centre (41.7272, 11.0721) ccw
  arc A282 (41.972, 26.583) -> (41.972, 25.083) centre (41.972, 25.833) ccw
  arc A283 (41.972, 26.583) -> (41.972, 25.083) centre (41.972, 25.833) ccw
  arc A284 (34.3063, 2.6578) -> (34.3063, 1.1578) centre (34.3063, 1.9078) ccw
  arc A285 (34.3063, 2.6578) -> (34.3063, 1.1578) centre (34.3063, 1.9078) ccw
  arc A286 (39.5249, 2.4663) -> (39.5249, 2.2377) centre (39.5249, 2.352) ccw
  arc A287 (10.6858, 8.7122) -> (10.6858, 8.9408) centre (10.6858, 8.8265) ccw
  arc A288 (39.5249, 2.4663) -> (39.5249, 2.2377) centre (39.5249, 2.352) ccw
  arc A289 (39.5249, 2.2377) -> (39.5249, 2.4663) centre (39.5249, 2.352) ccw
  arc A290 (10.6858, 8.9408) -> (10.6858, 8.7122) centre (10.6858, 8.8265) ccw
  arc A291 (21.6783, 12.2455) -> (21.6783, 12.4741) centre (21.6783, 12.3598) ccw
  arc A292 (21.6783, 12.2455) -> (21.6783, 12.4741) centre (21.6783, 12.3598) ccw
  arc A293 (21.6783, 12.4741) -> (21.6783, 12.2455) centre (21.6783, 12.3598) ccw
  arc A294 (21.6783, 11.6486) -> (21.6783, 11.8772) centre (21.6783, 11.7629) ccw
  arc A295 (21.6783, 12.4741) -> (21.6783, 12.2455) centre (21.6783, 12.3598) ccw
  arc A296 (21.6783, 11.8772) -> (21.6783, 11.6486) centre (21.6783, 11.7629) ccw
  arc A297 (21.6783, 11.8772) -> (21.6783, 11.6486) centre (21.6783, 11.7629) ccw
  arc A298 (21.6783, 11.6486) -> (21.6783, 11.8772) centre (21.6783, 11.7629) ccw
  arc A299 (20.7554, 19.4752) -> (20.7554, 19.7038) centre (20.7554, 19.5895) ccw
  arc A300 (20.7554, 19.4752) -> (20.7554, 19.7038) centre (20.7554, 19.5895) ccw
  arc A301 (20.7554, 19.7038) -> (20.7554, 19.4752) centre (20.7554, 19.5895) ccw
  arc A302 (20.7554, 19.7038) -> (20.7554, 19.4752) centre (20.7554, 19.5895) ccw
  arc A303 (22.3683, 14.6188) -> (22.3683, 14.8474) centre (22.3683, 14.7331) ccw
  arc A304 (22.3683, 14.6188) -> (22.3683, 14.8474) centre (22.3683, 14.7331) ccw
  arc A305 (22.3683, 14.8474) -> (22.3683, 14.6188) centre (22.3683, 14.7331) ccw
  arc A306 (22.3683, 14.8474) -> (22.3683, 14.6188) centre (22.3683, 14.7331) ccw
  arc A307 (23.6179, 10.9485) -> (23.6179, 11.1771) centre (23.6179, 11.0628) ccw
  arc A308 (23.6179, 10.9485) -> (23.6179, 11.1771) centre (23.6179, 11.0628) ccw
  arc A309 (23.6179, 11.1771) -> (23.6179, 10.9485) centre (23.6179, 11.0628) ccw
  arc A310 (23.6179, 11.1771) -> (23.6179, 10.9485) centre (23.6179, 11.0628) ccw
  arc A311 (35.6474, 26.1428) -> (35.6474, 26.3714) centre (35.6474, 26.2571) ccw
  arc A312 (35.6474, 26.1428) -> (35.6474, 26.3714) centre (35.6474, 26.2571) ccw
  arc A313 (35.6474, 26.3714) -> (35.6474, 26.1428) centre (35.6474, 26.2571) ccw
  arc A314 (35.6474, 26.3714) -> (35.6474, 26.1428) centre (35.6474, 26.2571) ccw
  arc A315 (35.6474, 25.4244) -> (35.6474, 25.653) centre (35.6474, 25.5387) ccw
  arc A316 (35.6474, 25.4244) -> (35.6474, 25.653) centre (35.6474, 25.5387) ccw
  arc A317 (35.6474, 25.653) -> (35.6474, 25.4244) centre (35.6474, 25.5387) ccw
  arc A318 (35.6474, 25.653) -> (35.6474, 25.4244) centre (35.6474, 25.5387) ccw
  arc A319 (35.6474, 24.7061) -> (35.6474, 24.9347) centre (35.6474, 24.8204) ccw
  arc A320 (35.6474, 24.7061) -> (35.6474, 24.9347) centre (35.6474, 24.8204) ccw
  arc A321 (35.6474, 24.9347) -> (35.6474, 24.7061) centre (35.6474, 24.8204) ccw
  arc A322 (35.6474, 24.9347) -> (35.6474, 24.7061) centre (35.6474, 24.8204) ccw
  arc A323 (35.6474, 23.9878) -> (35.6474, 24.2164) centre (35.6474, 24.1021) ccw
  arc A324 (35.6474, 23.9878) -> (35.6474, 24.2164) centre (35.6474, 24.1021) ccw
  arc A325 (35.6474, 24.2164) -> (35.6474, 23.9878) centre (35.6474, 24.1021) ccw
  arc A326 (35.6474, 24.2164) -> (35.6474, 23.9878) centre (35.6474, 24.1021) ccw
  arc A327 (17.5931, 13.8593) -> (17.5931, 14.0879) centre (17.5931, 13.9736) ccw
  arc A328 (17.5931, 13.8593) -> (17.5931, 14.0879) centre (17.5931, 13.9736) ccw
  arc A329 (17.5931, 14.0879) -> (17.5931, 13.8593) centre (17.5931, 13.9736) ccw
  arc A330 (13.0109, 8.3363) -> (13.0109, 8.5649) centre (13.0109, 8.4506) ccw
  arc A331 (17.5931, 14.0879) -> (17.5931, 13.8593) centre (17.5931, 13.9736) ccw
  arc A332 (13.0109, 8.5649) -> (13.0109, 8.3363) centre (13.0109, 8.4506) ccw
  arc A333 (13.0109, 8.5649) -> (13.0109, 8.3363) centre (13.0109, 8.4506) ccw
  arc A334 (13.0109, 8.3363) -> (13.0109, 8.5649) centre (13.0109, 8.4506) ccw
  arc A335 (18.383, 13.872) -> (18.383, 14.1006) centre (18.383, 13.9863) ccw
  arc A336 (18.383, 13.872) -> (18.383, 14.1006) centre (18.383, 13.9863) ccw
  arc A337 (18.383, 14.1006) -> (18.383, 13.872) centre (18.383, 13.9863) ccw
  arc A338 (13.4554, 7.9096) -> (13.4554, 8.1382) centre (13.4554, 8.0239) ccw
  arc A339 (18.383, 14.1006) -> (18.383, 13.872) centre (18.383, 13.9863) ccw
  arc A340 (13.4554, 8.1382) -> (13.4554, 7.9096) centre (13.4554, 8.0239) ccw
  arc A341 (13.4554, 8.1382) -> (13.4554, 7.9096) centre (13.4554, 8.0239) ccw
  arc A342 (13.4554, 7.9096) -> (13.4554, 8.1382) centre (13.4554, 8.0239) ccw
  arc A343 (19.0383, 6.4933) -> (19.0383, 6.7219) centre (19.0383, 6.6076) ccw
  arc A344 (19.0383, 6.4933) -> (19.0383, 6.7219) centre (19.0383, 6.6076) ccw
  arc A345 (19.0383, 6.7219) -> (19.0383, 6.4933) centre (19.0383, 6.6076) ccw
  arc A346 (19.0383, 6.7219) -> (19.0383, 6.4933) centre (19.0383, 6.6076) ccw
  arc A347 (23.9735, 10.1026) -> (23.9735, 10.3312) centre (23.9735, 10.2169) ccw
  arc A348 (23.9735, 10.1026) -> (23.9735, 10.3312) centre (23.9735, 10.2169) ccw
  arc A349 (23.9735, 10.3312) -> (23.9735, 10.1026) centre (23.9735, 10.2169) ccw
  arc A350 (23.9735, 10.3312) -> (23.9735, 10.1026) centre (23.9735, 10.2169) ccw
  arc A351 (26.0132, 11.4996) -> (26.0132, 11.7282) centre (26.0132, 11.6139) ccw
  arc A352 (26.0132, 11.4996) -> (26.0132, 11.7282) centre (26.0132, 11.6139) ccw
  arc A353 (26.0132, 11.7282) -> (26.0132, 11.4996) centre (26.0132, 11.6139) ccw
  arc A354 (26.0132, 11.7282) -> (26.0132, 11.4996) centre (26.0132, 11.6139) ccw
  arc A355 (22.7747, 12.0051) -> (22.7747, 12.2337) centre (22.7747, 12.1194) ccw
  arc A356 (22.7747, 12.0051) -> (22.7747, 12.2337) centre (22.7747, 12.1194) ccw
  arc A357 (22.7747, 12.2337) -> (22.7747, 12.0051) centre (22.7747, 12.1194) ccw
  arc A358 (22.7747, 12.2337) -> (22.7747, 12.0051) centre (22.7747, 12.1194) ccw
  arc A359 (21.8857, 10.476) -> (21.8857, 10.7046) centre (21.8857, 10.5903) ccw
  arc A360 (21.8857, 10.476) -> (21.8857, 10.7046) centre (21.8857, 10.5903) ccw
  arc A361 (21.8857, 10.7046) -> (21.8857, 10.476) centre (21.8857, 10.5903) ccw
  arc A362 (21.8857, 10.7046) -> (21.8857, 10.476) centre (21.8857, 10.5903) ccw
  arc A363 (21.111, 10.7757) -> (21.111, 11.0043) centre (21.111, 10.89) ccw
  arc A364 (21.111, 10.7757) -> (21.111, 11.0043) centre (21.111, 10.89) ccw
  arc A365 (21.111, 11.0043) -> (21.111, 10.7757) centre (21.111, 10.89) ccw
  arc A366 (21.111, 11.0043) -> (21.111, 10.7757) centre (21.111, 10.89) ccw
  arc A367 (22.7747, 10.6056) -> (22.7747, 10.8342) centre (22.7747, 10.7199) ccw
  arc A368 (22.7747, 10.6056) -> (22.7747, 10.8342) centre (22.7747, 10.7199) ccw
  arc A369 (22.7747, 10.8342) -> (22.7747, 10.6056) centre (22.7747, 10.7199) ccw
  arc A370 (22.7747, 10.8342) -> (22.7747, 10.6056) centre (22.7747, 10.7199) ccw
  arc A371 (24.004, 13.081) -> (24.004, 13.3096) centre (24.004, 13.1953) ccw
  arc A372 (24.004, 13.081) -> (24.004, 13.3096) centre (24.004, 13.1953) ccw
  arc A373 (24.004, 13.3096) -> (24.004, 13.081) centre (24.004, 13.1953) ccw
  arc A374 (24.9997, 10.2184) -> (24.9997, 10.447) centre (24.9997, 10.3327) ccw
  arc A375 (24.004, 13.3096) -> (24.004, 13.081) centre (24.004, 13.1953) ccw
  arc A376 (24.9997, 10.447) -> (24.9997, 10.2184) centre (24.9997, 10.3327) ccw
  arc A377 (24.9997, 10.447) -> (24.9997, 10.2184) centre (24.9997, 10.3327) ccw
  arc A378 (24.9997, 10.2184) -> (24.9997, 10.447) centre (24.9997, 10.3327) ccw
  arc A379 (23.1938, 11.5377) -> (23.1938, 11.7663) centre (23.1938, 11.652) ccw
  arc A380 (23.1938, 11.5377) -> (23.1938, 11.7663) centre (23.1938, 11.652) ccw
  arc A381 (23.1938, 11.7663) -> (23.1938, 11.5377) centre (23.1938, 11.652) ccw
  arc A382 (23.1938, 11.7663) -> (23.1938, 11.5377) centre (23.1938, 11.652) ccw
  arc A383 (22.3733, 15.4457) -> (22.3733, 15.6743) centre (22.3733, 15.56) ccw
  arc A384 (22.3733, 15.4457) -> (22.3733, 15.6743) centre (22.3733, 15.56) ccw
  arc A385 (22.3733, 15.6743) -> (22.3733, 15.4457) centre (22.3733, 15.56) ccw
  arc A386 (22.3733, 15.6743) -> (22.3733, 15.4457) centre (22.3733, 15.56) ccw
  arc A387 (23.1785, 15.4519) -> (23.1785, 15.6805) centre (23.1785, 15.5662) ccw
  arc A388 (23.1785, 15.4519) -> (23.1785, 15.6805) centre (23.1785, 15.5662) ccw